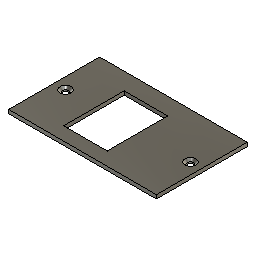
PSU_socket_holder_cover v3 (Autodesk Fusion 360 design; units mm, degrees)
Autodesk Fusion 360 part; units mm, degrees
sketch "Sketch1" plane through (0, 0, 0) normal (0, 0, 1) x (1, 0, 0)
  line L0 (0, 0) -> (78, 0)
  line L1 (78, 0) -> (78, 48)
  line L2 (78, 48) -> (0, 48)
  line L3 (0, 48) -> (0, 0)
  dimension "d1" = 78
  dimension "d2" = 48
  constraint horizontal L0
  constraint vertical L1
  constraint horizontal L2
  constraint vertical L3
  constraint coincident L0.start L3.end
  measures "d1" distance of L0.start L0.end
  measures "d2" distance of L0.start L2.end
extrude "Extrude1" add sketch "Sketch1" along normal blind 2
sketch "Sketch2" plane through (0, 0, 2) normal (0, 0, 1) x (-1, 0, 0)
  line L0 (0, -48) -> (0, 0)
  line L1 (0, 0) -> (-78, 0)
  line L2 (-78, 0) -> (-78, -48)
  line L3 (-78, -48) -> (0, -48)
  point P0 (-72, -24)
  point P1 (-6, -24)
hole "Hole1" at (72, 24, 2) at (6, 24, 2) direction (0, 0, -1) diameter 3.4 depth 13 tip angle 118 countersink diameter 5.8 countersink angle 90
sketch "Sketch3" plane through (0, 0, 2) normal (0, 0, 1) x (-1, 0, 0)
  circle A0 centre (-72, -24) radius 2.9
  circle A1 centre (-6, -24) radius 2.9
  line L0 (0, -48) -> (0, 0)
  line L1 (0, 0) -> (-78, 0)
  line L2 (-78, 0) -> (-78, -48)
  line L3 (-78, -48) -> (0, -48)
  line L4 (-22, -39) -> (-45, -39)
  line L5 (-45, -39) -> (-45, -7)
  line L6 (-45, -7) -> (-22, -7)
  line L7 (-22, -7) -> (-22, -39)
  constraint horizontal L4
  constraint vertical L5
  constraint horizontal L6
  constraint vertical L7
extrude "Extrude2" cut sketch "Sketch3" against normal blind 500 contours L4 L5 L6 L7
